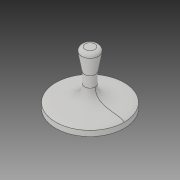
# Autodesk Inventor part: Top1
Saved by Autodesk Inventor 2018 (Build 220112000, 112)
## iProperties
Created: 2017-12-12
Part Number: Top1
Material: Generic
Document SubType Name: Modeling
Designer: Rus
Density: 1 g/cm^3
Appearance: Default
Author: Rus
Autodesk Inventor part; units mm, degrees
ref_plane "YZ Plane" through (0, 0, 0) normal (1, 0, 0) x (0, 1, 0)
ref_plane "XZ Plane" through (0, 0, 0) normal (0, 1, 0) x (-1, 0, 0)
ref_plane "XY Plane" through (0, 0, 0) normal (0, 0, 1) x (1, 0, 0)
sketch "Sketch1" plane through (0, 0, 0) normal (0, 0, 1) x (1, 0, 0)
  line L0 (0, 0) -> (0, 25.4)
  line L1 (0, 0) -> (0, -6.35)
  line L2 (0, 25.4) -> (0, 38.1)
  line L3 (5.4144, 38.1) -> (0, 38.1)
  line L4 (3.175, 16.8251) -> (0, 16.8251) construction
  line L5 (3.175, 25.4) -> (0, 25.4) construction
  line L6 (0, 0) -> (3.175, 0) construction
  line L7 (3.175, 0) -> (18.1464, 0) construction
  line L8 (0, -6.35) -> (3.175, -4.2333)
  line L9 (3.175, -4.2333) -> (3.175, 0)
  line L10 (3.175, 25.4) -> (3.175, 19.05)
  arc A0 (6.0772, 2.8494) -> (3.175, 0) centre (6.0248, 0) ccw
  line L11 (3.175, 19.05) -> (3.175, 9.1187) construction
  line L12 (3.175, 9.1187) -> (16.4968, 12.5871) construction
  line L13 (16.4968, 12.5871) -> (20.32, 9.525) construction
  spline S0 degree 3 poles (3.175, 19.05) (3.175, 9.1187) (16.4968, 12.5871) (20.32, 9.525) knots 1 1 1 1 2 2 2 2
  line L14 (6.0772, 2.8494) -> (16.4968, 2.658) construction
  line L15 (16.4968, 2.658) -> (20.32, 6.35) construction
  spline S1 degree 2 poles (6.0772, 2.8494) (16.4968, 2.658) (20.32, 6.35) knots 1 1 1 2 2 2
  line L16 (20.32, 6.35) -> (20.32, 9.525)
  line L17 (3.175, 25.4) -> (5.4144, 38.1)
  dimension "d5" = 44.45
  dimension "d12" = 2.1167
  dimension "d13" = 3.175
  dimension "d15" = 4.2333
  dimension "d31" = 6.35
  dimension "d33" = 20.32
  dimension "d34" = 6.35
  dimension "d35" = 3.175
  dimension "d37" = 10
  dimension "d38" = 3.175
  dimension "d39" = 12.7
  constraints: 27 end point, 7 vertical, 2 horizontal, 2 perpendicular, 2 point on circle, 2 point on line, 2 vertical alignment, 1 centre point, 1 tangent, 7 other
  measures "d5" distance of L2.end L1.end
  measures "d12" vertical distance of L8.end L1.end
  measures "d13" horizontal distance of L1.end L8.end
  measures "d15" distance from line of L7 L8.end
  measures "d31" distance of L5.start L10.end
  measures "d33" distance between parallel lines of L0 L16
  measures "d34" distance from line of L6 L15.end
  measures "d35" distance of L15.end L13.end
  measures "d37" angle of L10 L17
  measures "d38" distance between parallel lines of L0 L10
  measures "d39" distance from line of L3 L5.start
revolve "Revolution1" add sketch "Sketch1" angle 360 about axis through (0, 25.4, 0) along (0, -1, 0)
fillet "Fillet1" radius 2.1167 1 edges at (-5.4144, 38.1, 0)
body "Solid1"
